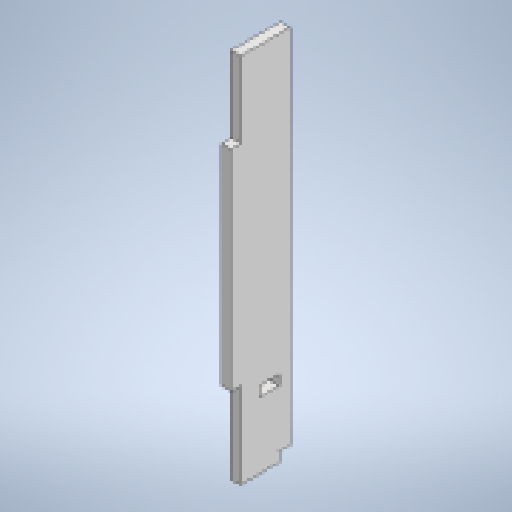
# Autodesk Inventor part: FanVerticalPlate
Saved by Autodesk Inventor 2023 (Build 270158000, 158)
## iProperties
Created: 2023-08-30
Part Number: FanVerticalPlate
Material: Generic
Document SubType Name: Modeling
Designer: Nathann
Density: 1 g/cm^3
Appearance: Default
Author: Nathann
Autodesk Inventor part; units mm, degrees
ref_plane "YZ Plane" through (0, 0, 0) normal (1, 0, 0) x (0, 1, 0)
ref_plane "XZ Plane" through (0, 0, 0) normal (0, 1, 0) x (-1, 0, 0)
ref_plane "XY Plane" through (0, 0, 0) normal (0, 0, 1) x (1, 0, 0)
sketch "Sketch1" plane through (0, 0, 0) normal (1, 0, 0) x (0, 1, 0)
  line L0 (0, 0) -> (200, 0)
  line L1 (200, 0) -> (200, 31)
  line L2 (200, 31) -> (0, 31)
  line L3 (0, 31) -> (0, 0)
  dimension "d0" = 31
  dimension "d1" = 200
  constraints: 8 end point, 2 parallel, 1 horizontal, 1 perpendicular
  measures "d0" distance between parallel lines of L0 L2
  measures "d1" distance of L1.end L2.end
extrude "Extrusion1" add sketch "Sketch1" along normal blind 5
sketch "Sketch2" plane through (0, 0, 0) normal (-1, 0, 0) x (0, 0, 1)
  line L0 (0, 200) -> (31, 200) projected
  line L1 (31, 200) -> (26, 200)
  line L2 (26, 200) -> (26, 195)
  line L3 (26, 195) -> (31, 195)
  line L4 (31, 195) -> (31, 200)
  line L5 (0, 200) -> (5, 200)
  line L6 (5, 200) -> (5, 195)
  line L7 (5, 195) -> (0, 195)
  line L8 (0, 195) -> (0, 200)
  line L9 (31, 0) -> (0, 0) projected
  line L10 (0, 0) -> (5, 0)
  line L11 (5, 0) -> (5, 5)
  line L12 (5, 5) -> (0, 5)
  line L13 (0, 5) -> (0, 0)
  line L14 (31, 200) -> (31, 0) projected
  line L15 (31, 0) -> (26, 0)
  line L16 (26, 0) -> (26, 5)
  line L17 (26, 5) -> (31, 5)
  line L18 (31, 5) -> (31, 0)
  line L19 (31, 195) -> (26, 195)
  line L20 (26, 195) -> (26, 155)
  line L21 (26, 155) -> (31, 155)
  line L22 (31, 155) -> (31, 195)
  line L23 (31, 5) -> (26, 5)
  line L24 (26, 5) -> (26, 45)
  line L25 (26, 45) -> (31, 45)
  line L26 (31, 45) -> (31, 5)
  point P0 (31, 5)
  point P1 (26, 0)
  point P2 (31, 45)
  point P3 (31, 155)
  dimension "d4" = 5
  dimension "d5" = 5
  dimension "d6" = 5
  dimension "d7" = 5
  dimension "d8" = 5
  dimension "d9" = 5
  dimension "d10" = 5
  dimension "d11" = 5
  dimension "d14" = 40
  dimension "d15" = 40
  constraints: 48 end point, 12 parallel, 6 horizontal, 6 perpendicular, 2 point on line
  measures "d4" distance of L10.end L11.end
  measures "d5" distance of L11.end L12.end
  measures "d6" distance of L15.end L16.end
  measures "d7" distance of L16.end L17.end
  measures "d8" distance of L6.end L7.end
  measures "d9" distance of L5.end L6.end
  measures "d10" distance of L1.end L2.end
  measures "d11" distance of L2.end L3.end
  measures "d14" distance of L19.end L20.end
  measures "d15" distance of L23.end L24.end
extrude "Extrusion2" cut sketch "Sketch2" against normal blind 10 contours L0 L4 L3 L2 | L3 L14 L21 L20 | L9 L16 L17 L14 | L17 L24 L25 L14
sketch "Sketch3" plane through (0, 0, 0) normal (-1, 0, 0) x (0, 0, 1)
  line L0 (6, 35) -> (16, 35) projected
  line L1 (6, 40) -> (16, 40) projected
  line L2 (1, 40) -> (1, 35) projected
  line L3 (16, 40) -> (16, 35)
  line L4 (26, 45) -> (26, 0) projected
  point P0 (0, 0)
  point P1 (26, 0)
  constraints: 2 end point, 1 vertical, 1 other
sketch "Sketch3 outline for Extrusion3" plane through (0, 0, 0) normal (-1, 0, 0) x (0, 0, 1)
  line L0 (6, 40) -> (6, 35)
  line L1 (16, 40) -> (6, 40)
  line L2 (16, 35) -> (16, 40)
  line L3 (6, 35) -> (16, 35)
extrude "Extrusion3" cut sketch "Sketch3 outline for Extrusion3" against normal blind 10
sketch "Sketch4" plane through (0, 0, 0) normal (-1, 0, 0) x (0, 0, 1)
  line L0 (26, 200) -> (26, 155) projected
  line L1 (0, 0) -> (0, 200) projected
  line L2 (26, 200) -> (0, 200)
  line L3 (0, 200) -> (0, 195)
  line L4 (0, 195) -> (26, 195)
  line L5 (26, 195) -> (26, 200)
  dimension "d18" = 5
  constraints: 8 end point, 2 parallel, 1 horizontal, 1 perpendicular, 1 point on line
  measures "d18" distance between parallel lines of L2 L4
extrude "Extrusion4" cut sketch "Sketch4" against normal blind 10
sketch "Sketch5" plane through (5, 0, 0) normal (1, 0, 0) x (0, 0, -1)
  line L0 (0, 0) -> (0, 195) projected
  line L1 (0, 0) -> (-6, 0)
  line L2 (-6, 0) -> (-6, 5)
  line L3 (-6, 5) -> (0, 5)
  line L4 (0, 5) -> (0, 0)
  line L5 (-6, 40) -> (-6, 35) projected
  point P0 (0, 5)
  dimension "d21" = 6
  dimension "d22" = 5
  dimension "d23" = 6
  constraints: 8 end point, 2 parallel, 1 horizontal, 1 perpendicular
  measures "d21" distance of L2.end L3.end
  measures "d22" distance of L1.end L2.end
  measures "d23" distance between parallel lines of L0 L5
extrude "Extrusion5" cut sketch "Sketch5" against normal blind 10
equation "\"d6\" = d4"
equation "\"d7\" = d4"
equation "\"d8\" = d5"
equation "\"d9\" = d8"
equation "\"d11\" = d8"
body "Solid1"
